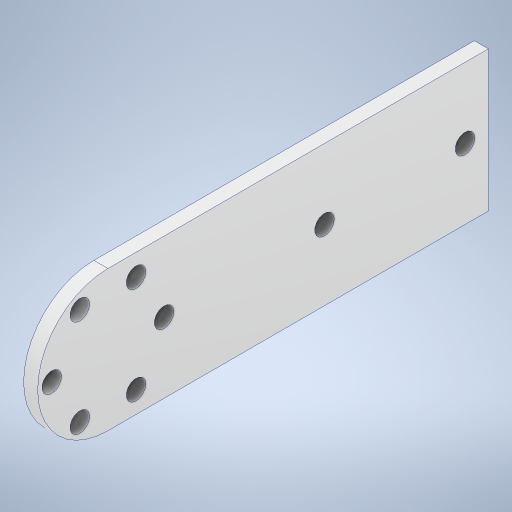
# Autodesk Inventor part: link4_plate4
Saved by Autodesk Inventor 2024 (Build 280153000, 153)
## iProperties
Created: 2024-12-13
Part Number: link4_plate4
Material: アルミニウム 6061
Document SubType Name: Modeling
Designer: hirek
Density: 2.7 g/cm^3
Appearance: アルミニウム - フラット
Mass: 37.9594 g
Surface Area: 106.915 cm^2
Volume: 14.059 cm^3
Author: hirek
Autodesk Inventor part; units mm, degrees
ref_plane "YZ Plane" through (0, 0, 0) normal (1, 0, 0) x (0, 1, 0)
ref_plane "XZ Plane" through (0, 0, 0) normal (0, 1, 0) x (-1, 0, 0)
ref_plane "XY Plane" through (0, 0, 0) normal (0, 0, 1) x (1, 0, 0)
sketch "スケッチ1" plane through (0, 0, 0) normal (1, 0, 0) x (0, 1, 0)
  circle A0 centre (0, 0) radius 15
  line L0 (15, -41.25) -> (-15, -41.25)
  line L1 (-15, -41.25) -> (-15, -81.25)
  line L2 (-15, -81.25) -> (15, -81.25)
  line L3 (15, -81.25) -> (15, -41.25)
  line L4 (15, -41.25) -> (15, 0)
  line L5 (-15, 0) -> (-15, -41.25)
  dimension "d0" = 30
  dimension "d1" = 30
  dimension "d2" = 40
  dimension "d4" = 15
  dimension "d28" = 41.25
  constraints: 12 end point, 2 parallel, 2 point on circle, 2 tangent, 1 centre point, 1 coincident, 1 horizontal, 1 perpendicular
  measures "d0" diameter of A0
  measures "d1" distance of L2.end L1.end
  measures "d2" distance of L1.end L0.end
  measures "d4" distance from line of L3 point (0, 0)
  measures "d28" distance from line of L0 point (0, 0)
extrude "押し出し1" add sketch "スケッチ1" along normal blind 3
sketch "スケッチ2" plane through (3, 0, 0) normal (1, 0, 0) x (0, 0, -1)
  circle A0 centre (0, 0) radius 12
  line L0 (81.25, 15) -> (0, 15) projected
  line L1 (81.25, -15) -> (81.25, 15) projected
  point P0 (12, 0)
  point P1 (6, 10.3923)
  point P2 (-6, 10.3923)
  point P3 (-12, 0)
  point P4 (-6, -10.3923)
  point P5 (6, -10.3923)
  dimension "d7" = 24
  dimension "d10" = 360
  constraints: 1 coincident, 1 horizontal alignment, 9 other
hole "穴1" at (3, 0, -12) at (3, 10.3923, -6) at (3, 10.3923, 6) at (3, 0, 12) at (3, -10.3923, 6) at (3, -10.3923, -6) direction (-1, 0, 0) diameter 4.2 end through all
sketch "スケッチ5" plane through (3, 0, 0) normal (1, 0, 0) x (0, 0, -1)
  line L0 (81.25, -15) -> (81.25, 15) projected
  point P0 (0, 0)
  point P1 (76.25, 0)
  point P2 (46.25, 0)
  dimension "d40" = 5
  dimension "d41" = 30
  measures "d40" distance from line of point (76.25, 0) L0
  measures "d41" distance of point (46.25, 0) point (76.25, 0)
hole "穴3" at (3, 0, -76.25) at (3, 0, -46.25) direction (-1, 0, 0) diameter 4.2 end through all
